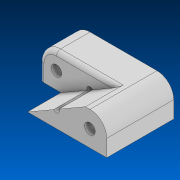
# Autodesk Inventor part: Intake Stopper
Saved by Autodesk Inventor 2022.2 (Build 262287000, 287)
## iProperties
Created: 2022-04-25
Part Number: Intake Stopper
Material: Generic
Document SubType Name: Modeling
Designer: omard
Density: 1 g/cm^3
Appearance: Default
Author: omard
Autodesk Inventor part; units mm, degrees
ref_plane "YZ Plane" through (0, 0, 0) normal (1, 0, 0) x (0, 1, 0)
ref_plane "XZ Plane" through (0, 0, 0) normal (0, 1, 0) x (-1, 0, 0)
ref_plane "XY Plane" through (0, 0, 0) normal (0, 0, 1) x (1, 0, 0)
sketch "Sketch1" plane through (0, 0, 0) normal (0, 0, 1) x (1, 0, 0)
  line L0 (-38.1, 12.7) -> (38.1, 12.7)
  line L1 (38.1, 12.7) -> (38.1, -12.7)
  line L2 (38.1, -12.7) -> (-38.1, -12.7)
  line L3 (-38.1, -12.7) -> (-38.1, 12.7)
  line L4 (-38.1, 12.7) -> (38.1, -12.7) construction
  line L5 (38.1, 12.7) -> (-38.1, -12.7) construction
  line L6 (21.997, 12.7) -> (-21.997, -12.7)
  point P0 (0, 0)
  point P1 (25.4, 0)
  point P2 (0, 0)
  point P3 (-25.4, 0)
  point P4 (0, 0)
  point P5 (0, 0)
  dimension "d0" = 25.4
  dimension "d1" = 25.4
  dimension "d2" = 25.4
  dimension "d3" = 12.7
  dimension "d4" = 30
  constraints: 14 end point, 5 midpoint, 2 horizontal alignment, 2 parallel, 2 point on line, 1 coincident, 1 horizontal, 1 perpendicular
  measures "d0" distance between parallel lines of L2 L0
  measures "d1" distance of point (0, 0) point (-25.4, 0)
  measures "d2" distance of point (0, 0) point (25.4, 0)
  measures "d3" distance from line of L3 point (-25.4, 0)
  measures "d4" angle of L0 L6
extrude "Extrusion1" add sketch "Sketch1" against normal blind 25.4
extrude "Extrusion2" add sketch "Sketch1" along normal blind 25.4 contours L0 L1 L2 L6
hole "Hole1" at (25.4, 0, 0) at (0, 0, 0) at (-25.4, 0, 0) direction (0, 0, 1) diameter 4.445 end through all start extended yes
hole "Hole2" at (-25.4, 0, 0) at (25.4, 0, 0) direction (0, 0, -1) diameter 4.445 end through all start extended yes counterbore diameter 8.001 counterbore depth 12.7
fillet "Fillet2" radius 12.7 2 edges at (-38.1, 12.7, -12.7) (38.1, 12.7, 0)
fillet "Fillet1" radius 3.175 1 edges at (-1.7015, 12.7, 0)
sketch "Sketch2" plane through (0, 0, -25.4) normal (0, 0, -1) x (-1, 0, 0)
  circle A0 centre (0, 0) radius 2.2225 projected
  constraints: 1 coincident
hole "Hole3" at (0, 0, -25.4) direction (0, 0, 1) diameter 4.445 end through all start extended yes counterbore diameter 8.001 counterbore depth 3.81
body "Solid1"
